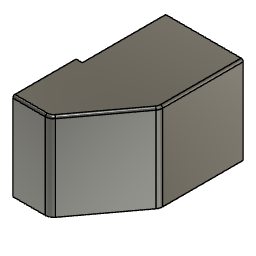
왼쪽 사이드 범퍼 (Autodesk Fusion 360 design; units mm, degrees)
Autodesk Fusion 360 part; units mm, degrees
sketch "스케치1" plane through (0, 0, 0) normal (0, 0, 1) x (1, 0, 0)
  line L0 (0, 0) -> (44, 0)
  line L1 (0, 0) -> (0, 4)
  line L2 (0, 4) -> (41, 4)
  line L3 (0, 0) -> (44, 0)
  line L4 (44, 0) -> (100.5, 76)
  line L5 (100.5, 76) -> (97.5, 76)
  line L6 (44, 0) -> (41, 0)
  line L7 (41, 0) -> (97.5, 76)
  line L8 (41, 4) -> (43.9737, 4)
  line L9 (100.5, 76) -> (97.5, 76)
  line L10 (97.5, 76) -> (97.5, 176)
  line L11 (97.5, 176) -> (100.5, 176)
  line L12 (100.5, 176) -> (100.5, 76)
  line L13 (0, 4) -> (0, 76)
  line L14 (0, 76) -> (7.5, 76)
  line L15 (7.5, 76) -> (12.5, 76)
  line L16 (12.5, 76) -> (12.5, 96)
  line L17 (12.5, 96) -> (7.5, 96)
  line L18 (7.5, 96) -> (7.5, 76)
  line L19 (97.5, 176) -> (12.5, 176)
  line L20 (12.5, 176) -> (12.5, 173)
  line L21 (12.5, 173) -> (97.5, 173)
  line L22 (97.5, 173) -> (97.5, 176)
  line L23 (12.5, 176) -> (7.5, 176)
  line L24 (7.5, 176) -> (7.5, 153)
  line L25 (7.5, 153) -> (12.5, 153)
  line L26 (12.5, 153) -> (12.5, 176)
  dimension "d1" = 44
  dimension "d2" = 4
  dimension "d3" = 41
  dimension "d7" = 3
  dimension "d8" = 3
  dimension "d9" = 3
  dimension "d10" = 100
  dimension "d19" = 72
  dimension "d20" = 7.5
  dimension "d21" = 5
  dimension "d22" = 20
  dimension "d26" = 85
  dimension "d27" = 3
  dimension "d28" = 23
  constraint coincident L0.start L1.start
  constraint horizontal L0
  constraint perpendicular L0 L1
  constraint perpendicular L1 L2
  constraint perpendicular L1 L3
  constraint parallel L0 L6
  constraint coincident L7 L8.end
  constraint parallel L2 L8
  constraint horizontal L9
  constraint vertical L10
  constraint horizontal L11
  constraint vertical L12
  constraint perpendicular L2 L13
  constraint perpendicular L13 L14
  constraint horizontal L15
  constraint vertical L16
  constraint horizontal L17
  constraint vertical L18
  constraint horizontal L19
  constraint vertical L20
  constraint horizontal L21
  constraint vertical L22
  constraint horizontal L23
  constraint vertical L24
  constraint horizontal L25
  constraint vertical L26
  measures "d1" distance of L0.start L0.end
  measures "d2" distance of L0.start L1.end
  measures "d3" distance of L1.end L2.end
  measures "d7" distance of L4.end L5.end
  measures "d8" distance of L0.end L6.end
  measures "d9" distance of L4.end L5.end
  measures "d10" distance of L4.end L11.end
  measures "d19" distance of L1.end L13.end
  measures "d20" distance of L13.end L14.end
  measures "d21" distance of L14.end L15.end
  measures "d22" distance of L14.end L17.end
  measures "d26" distance of L10.end L19.end
  measures "d27" distance of L10.end L21.end
  measures "d28" distance of L19.end L25.end
extrude "돌출1" add sketch "스케치1" along normal blind 105 makes body 1 at (100.5, 142.6667, 35) makes body 2 at (7.5, 89.3333, 35)
sketch "스케치2" plane through (0, 0, 105) normal (0, 0, 1) x (-1, 0, 0)
  line L0 (0, 0) -> (-44, 0)
  line L1 (-44, 0) -> (-100.5, -76)
  line L2 (-100.5, -76) -> (-100.5, -176)
  line L3 (-100.5, -176) -> (-7.5, -176)
  line L4 (-97.5, -173) -> (-97.5, -76)
  line L5 (-97.5, -76) -> (-43.9737, -4)
  line L6 (-43.9737, -4) -> (0, -4)
  line L7 (0, -4) -> (0, 0)
  line L8 (0, -4) -> (0, -176)
  line L9 (0, -176) -> (-7.5, -176)
  line L10 (-12.5, -153) -> (-12.5, -173)
  line L11 (-12.5, -173) -> (-97.5, -173)
  line L12 (-7.5, -176) -> (-7.5, -153)
  line L13 (-7.5, -153) -> (-12.5, -153)
  constraint coincident L6.end L7.start
  constraint perpendicular L3 L8
  constraint coincident L3.end L9.end
  constraint perpendicular L4 L9
extrude "돌출2" add sketch "스케치2" against normal blind 3 contours L4 L5 L6 L8 L9 L10 L11 L12 L13 bodies 1 2
fillet "필렛1" radius 10 2 edges at (100.5, 76, 52.5) (44, 0, 52.5) on bodies 1
fillet "필렛2" radius 2.5 5 edges at (19.4868, 0, 105) (43.4646, 1.0652, 105) (72.7621, 38.6888, 105) (99.9935, 76.1676, 105) (100.5, 127.6549, 105) on bodies 1
sketch "스케치3" plane through (0, 173, 0) normal (0, -1, 0) x (1, 0, 0)
  line L0 (97.5, 102) -> (12.5, 102)
  line L1 (12.5, 102) -> (12.5, 0)
  line L2 (12.5, 0) -> (97.5, 0)
  line L3 (97.5, 0) -> (97.5, 102)
  line L4 (97.5, 0) -> (94.5, 0)
  line L5 (94.5, 0) -> (94.5, 3)
  line L6 (94.5, 3) -> (97.5, 3)
  line L7 (97.5, 3) -> (97.5, 0)
  line L8 (12.5, 102) -> (15.5, 102)
  line L9 (15.5, 102) -> (15.5, 99)
  line L10 (15.5, 99) -> (12.5, 99)
  line L11 (12.5, 99) -> (12.5, 102)
  line L12 (15.5, 99) -> (94.5, 99)
  line L13 (94.5, 99) -> (94.5, 3)
  line L14 (94.5, 3) -> (15.5, 3)
  line L15 (15.5, 3) -> (15.5, 99)
  line L16 (94.5, 99) -> (94.5, 56)
  line L17 (94.5, 56) -> (84.5, 56)
  line L18 (84.5, 56) -> (84.5, 46)
  line L19 (84.5, 46) -> (94.5, 46)
  line L20 (94.5, 46) -> (94.5, 56)
  line L21 (15.5, 56) -> (25.5, 56)
  line L22 (25.5, 56) -> (25.5, 46)
  line L23 (25.5, 46) -> (15.5, 46)
  line L24 (15.5, 46) -> (15.5, 56)
  circle A0 centre (89.5, 51) radius 2.15
  circle A1 centre (20.5, 51) radius 2.15
  dimension "d29" = 3
  dimension "d30" = 3
  dimension "d31" = 3
  dimension "d32" = 3
  dimension "d35" = 43
  dimension "d36" = 10
  dimension "d37" = 10
  dimension "d38" = 10
  dimension "d39" = 10
  dimension "d40" = 4.3
  dimension "d41" = 4.3
  constraint horizontal L4
  constraint vertical L5
  constraint horizontal L6
  constraint vertical L7
  constraint coincident L2.end L3.start
  constraint horizontal L8
  constraint vertical L9
  constraint horizontal L10
  constraint vertical L11
  constraint coincident L0.end L1.start
  constraint horizontal L12
  constraint vertical L13
  constraint horizontal L14
  constraint vertical L15
  constraint perpendicular L6 L16
  constraint horizontal L17
  constraint vertical L18
  constraint horizontal L19
  constraint vertical L20
  constraint horizontal L21
  constraint vertical L22
  constraint horizontal L23
  constraint vertical L24
  constraint coincident L15 L21.start
  measures "d29" distance of L2.end L4.end
  measures "d30" distance of L2.end L6.end
  measures "d31" distance of L0.end L8.end
  measures "d32" distance of L0.end L10.end
  measures "d35" distance of L12.end L16.end
  measures "d36" distance of L16.end L17.end
  measures "d37" distance of L16.end L19.end
  measures "d38" distance of L21.start L21.end
  measures "d39" distance of L21.start L23.end
  measures "d40" diameter of A0
  measures "d41" diameter of A1
extrude "돌출3" cut sketch "스케치3" against normal blind 3 contours L12 L13 L14 L15 L16 L17 L18 L19 L21 L22 L23 | A0 | A1 bodies 1
sketch "스케치4" plane through (7.5, 0, 0) normal (-1, 0, 0) x (0, -1, 0)
  line L0 (-153, 102) -> (-176, 102)
  line L1 (-176, 102) -> (-176, 0)
  line L2 (-176, 0) -> (-153, 0)
  line L3 (-153, 0) -> (-153, 102)
  line L4 (-153, 102) -> (-153, 73)
  line L5 (-153, 73) -> (-173, 73)
  line L6 (-173, 73) -> (-173, 53)
  line L7 (-173, 53) -> (-153, 53)
  line L8 (-153, 53) -> (-153, 73)
  circle A0 centre (-163, 63) radius 2.65
  dimension "d42" = 29
  dimension "d43" = 20
  dimension "d44" = 20
  dimension "d45" = 5.3
  constraint coincident L0.start L3.end
  constraint perpendicular L0 L4
  constraint horizontal L5
  constraint vertical L6
  constraint horizontal L7
  constraint vertical L8
  measures "d42" distance of L0.start L4.end
  measures "d43" distance of L4.end L5.end
  measures "d44" distance of L4.end L7.end
  measures "d45" diameter of A0
sketch "스케치5" plane through (7.5, 0, 0) normal (-1, 0, 0) x (0, -1, 0)
  line L0 (-76, 102) -> (-96, 102)
  line L1 (-96, 102) -> (-96, 0)
  line L2 (-96, 0) -> (-76, 0)
  line L3 (-76, 0) -> (-76, 102)
  line L4 (-76, 102) -> (-76, 53)
  line L5 (-76, 53) -> (-96, 53)
  line L6 (-96, 53) -> (-96, 33)
  line L7 (-96, 33) -> (-76, 33)
  line L8 (-76, 33) -> (-76, 53)
  circle A0 centre (-86, 43) radius 2.65
  dimension "d46" = 49
  dimension "d47" = 20
  dimension "d48" = 5.3
  constraint coincident L0.start L3.end
  constraint perpendicular L0 L4
  constraint horizontal L5
  constraint vertical L6
  constraint horizontal L7
  constraint vertical L8
  measures "d46" distance of L0.start L4.end
  measures "d47" distance of L4.end L7.end
  measures "d48" diameter of A0
extrude "돌출4" cut sketch "스케치4" sketch "스케치5" against normal blind 5 contours A0 of sketch 2 contours A0 bodies 1
sketch "스케치6" plane through (0, 0, 102) normal (0, 0, -1) x (1, 0, 0)
  line L0 (7.5, -176) -> (7.5, -153)
  line L1 (7.5, -153) -> (12.5, -153)
  line L2 (12.5, -153) -> (12.5, -173)
  line L3 (12.5, -173) -> (97.5, -173)
  line L4 (97.5, -173) -> (97.5, -76)
  line L5 (97.5, -76) -> (43.9737, -4)
  line L6 (43.9737, -4) -> (0, -4)
  line L7 (0, -4) -> (0, -176)
  line L8 (0, -176) -> (7.5, -176)
  line L9 (12.5, -96) -> (7.5, -96)
  line L10 (7.5, -96) -> (7.5, -76)
  line L11 (7.5, -76) -> (12.5, -76)
  line L12 (12.5, -76) -> (12.5, -96)
  line L13 (0, -76) -> (7.5, -76)
  line L14 (7.5, -76) -> (7.5, -176)
  line L15 (7.5, -176) -> (0, -176)
  line L16 (0, -176) -> (0, -76)
  constraint horizontal L13
  constraint vertical L14
  constraint horizontal L15
  constraint vertical L16
  constraint coincident L0.start L8.end
  constraint coincident L7 L13.start
extrude "돌출5" cut sketch "스케치6" against normal blind 3 contours L0 L7 L8 L10 L13 L14 L15 L16 bodies 1
sketch "스케치7" plane through (0, 4, 0) normal (0, 1, 0) x (-1, 0, 0)
  line L0 (0, 102) -> (-43.9737, 102)
  line L1 (-43.9737, 102) -> (-43.9737, 0)
  line L2 (-43.9737, 0) -> (0, 0)
  line L3 (0, 0) -> (0, 102)
  line L4 (0, 0) -> (0, 28)
  line L5 (0, 28) -> (-3, 28)
  line L6 (-3, 28) -> (-3, 38)
  line L7 (-3, 38) -> (0, 38)
  line L8 (0, 38) -> (0, 28)
  dimension "d53" = 28
  dimension "d54" = 3
  dimension "d55" = 10
  constraint coincident L2.end L3.start
  constraint perpendicular L2 L4
  constraint horizontal L5
  constraint vertical L6
  constraint horizontal L7
  constraint vertical L8
  measures "d53" distance of L2.end L4.end
  measures "d54" distance of L4.end L5.end
  measures "d55" distance of L4.end L7.end
extrude "돌출6" add sketch "스케치7" along normal blind 13 contours L3 L5 L6 L7 L8 bodies 1
sketch "스케치8" plane through (0, 0, 0) normal (-1, 0, 0) x (0, -1, 0)
  line L0 (-76, 105) -> (-76, 102)
  line L1 (-76, 102) -> (-4, 102)
  line L2 (-4, 102) -> (-4, 38)
  line L3 (-4, 38) -> (-17, 38)
  line L4 (-17, 38) -> (-17, 28)
  line L5 (-17, 28) -> (-4, 28)
  line L6 (-4, 28) -> (-4, 0)
  line L7 (-4, 0) -> (0, 0)
  line L8 (0, 0) -> (0, 102.5)
  arc A0 (0, 102.5) -> (-2.5, 105) centre (-2.5, 102.5) ccw
  line L9 (-2.5, 105) -> (-76, 105)
  line L10 (-17, 38) -> (-7, 38)
  line L11 (-7, 38) -> (-7, 28)
  line L12 (-7, 28) -> (-17, 28)
  line L13 (-17, 28) -> (-17, 38)
  circle A1 centre (-12, 33) radius 2.15
  dimension "d58" = 4.3
  constraint horizontal L10
  constraint vertical L11
  constraint horizontal L12
  constraint vertical L13
  constraint coincident L5 L11.end
  constraint coincident L3.end L4.start
  measures "d58" diameter of A1
extrude "돌출7" cut sketch "스케치8" against normal blind 3 contours A1 bodies 1
sketch "스케치9" plane through (0, 0, 102) normal (0, 0, -1) x (1, 0, 0)
  line L0 (7.5, -96) -> (7.5, -153)
  line L1 (7.5, -153) -> (12.5, -153)
  line L2 (12.5, -153) -> (12.5, -173)
  line L3 (12.5, -173) -> (97.5, -173)
  line L4 (97.5, -173) -> (97.5, -76)
  line L5 (97.5, -76) -> (43.9737, -4)
  line L6 (43.9737, -4) -> (0, -4)
  line L7 (0, -4) -> (0, -76)
  line L8 (0, -76) -> (7.5, -76)
  line L9 (7.5, -76) -> (12.5, -76)
  line L10 (12.5, -76) -> (12.5, -96)
  line L11 (12.5, -96) -> (7.5, -96)
  line L12 (0, -4) -> (3, -4)
  line L13 (3, -4) -> (3, -10)
  line L14 (3, -10) -> (0, -10)
  line L15 (0, -10) -> (0, -4)
  dimension "d61" = 3
  dimension "d62" = 6
  constraint horizontal L12
  constraint vertical L13
  constraint horizontal L14
  constraint vertical L15
  constraint coincident L6.end L7.start
  measures "d61" distance of L6.end L12.end
  measures "d62" distance of L6.end L14.end
extrude "돌출8" add sketch "스케치9" along normal blind 64 contours L6 L7 L12 L13 L14 L15 bodies 1
sketch "스케치10" plane through (0, 0, 28) normal (0, 0, -1) x (1, 0, 0)
  line L0 (3, -4) -> (0, -4)
  line L1 (0, -4) -> (0, -17)
  line L2 (0, -17) -> (3, -17)
  line L3 (3, -17) -> (3, -4)
  line L4 (0, -4) -> (3, -4)
  line L5 (3, -4) -> (3, -10)
  line L6 (3, -10) -> (0, -10)
  line L7 (0, -10) -> (0, -4)
  dimension "d65" = 6
  constraint horizontal L4
  constraint vertical L5
  constraint horizontal L6
  constraint vertical L7
  constraint coincident L0.end L1.start
  measures "d65" distance of L0.end L6.end
extrude "돌출9" add sketch "스케치10" along normal blind 28 contours L0 L1 L3 L4 L5 L6 L7 bodies 1
